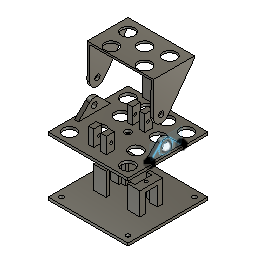
tableXY v18 (Autodesk Fusion 360 design; units mm, degrees)
Autodesk Fusion 360 part; units mm, degrees
sketch "Esquisse2" plane through (0, 0, 0) normal (0, 0, 1) x (1, 0, 0)
  line L0 (-25, 25) -> (25, 25)
  line L1 (25, 25) -> (25, -25)
  line L2 (25, -25) -> (-25, -25)
  line L3 (-25, -25) -> (-25, 25)
  line L4 (-25, 25) -> (25, -25) construction
  line L5 (25, 25) -> (-25, -25) construction
  circle A0 centre (-15.6977, 15.6977) radius 5
  circle A1 centre (-15.6977, -15.6977) radius 5
  circle A2 centre (15.6977, -15.6977) radius 5
  circle A3 centre (15.6977, 15.6977) radius 5
  circle A4 centre (-12.5, 0) radius 5
  circle A5 centre (0, -12.5) radius 5
  circle A6 centre (12.5, 0) radius 5
  circle A7 centre (0, 12.5) radius 5
  dimension "d1" = 50
  dimension "d2" = 50
  dimension "d3" = 10
  dimension "d9" = 360
  dimension "d11" = 10
  dimension "d13" = 360
  constraint horizontal L0
  constraint perpendicular L0 L1
  constraint parallel L0 L2
  constraint parallel L1 L3
  constraint coincident L4 origin
  constraint coincident L5 origin
  constraint coincident L4 A0.centre
  measures "d1" distance of L1.end L2.end
  measures "d2" distance of L0.end L1.end
  measures "d3" diameter of A0
  measures "d11" diameter of A4
extrude "Extrusion1" add sketch "Esquisse2" along normal blind 1.5 makes body 1
sketch "Esquisse3" plane through (0, 0, 0) normal (0, 0, -1) x (1, 0, 0)
  circle A0 centre (-12.5, 0) radius 5
  circle A1 centre (-15.6977, 15.6977) radius 5
  circle A2 centre (15.6977, 15.6977) radius 5
  circle A3 centre (15.6977, -15.6977) radius 5
  circle A4 centre (12.5, 0) radius 5
  circle A5 centre (0, -12.5) radius 5
  circle A6 centre (0, 12.5) radius 5
  circle A7 centre (-15.6977, -15.6977) radius 5
  line L0 (25, 25) -> (-25, 25)
  line L1 (-25, 25) -> (-25, -25)
  line L2 (-25, -25) -> (25, -25)
  line L3 (25, -25) -> (25, 25)
  line L4 (-25, -25) -> (-23, -25)
  line L5 (-23, -25) -> (-23, 25)
  line L6 (-23, 25) -> (-25, 25)
  line L7 (-25, 25) -> (-25, -25)
  line L8 (23, -25) -> (25, -25)
  line L9 (25, -25) -> (25, 25)
  line L10 (25, 25) -> (23, 25)
  line L11 (23, 25) -> (23, -25)
  dimension "d16" = 2
  dimension "d69" = 2
  constraint horizontal L4
  constraint vertical L5
  constraint horizontal L6
  constraint vertical L7
  constraint coincident L1.end L2.start
  constraint horizontal L8
  constraint vertical L9
  constraint horizontal L10
  constraint vertical L11
  constraint coincident L0.start L3.end
  constraint coincident L2 L8.start
  measures "d16" distance of L1.end L4.end
  measures "d69" distance of L9 L11
extrude "Extrusion2" add sketch "Esquisse3" along normal blind 30 contours L0 L2 L3 L8 L9 L10 L11 | L0 L1 L2 L4 L5 L6 L7 bodies 1
sketch "Esquisse4" plane through (-25, 0, 0) normal (-1, 0, 0) x (0, -1, 0)
  line L0 (25, -30) -> (25, 1.5)
  line L1 (25, 1.5) -> (-25, 1.5)
  line L2 (-25, 1.5) -> (-25, -30)
  line L3 (-25, -30) -> (25, -30)
  circle A0 centre (-0.0292, -23.958) radius 5.85
  circle A1 centre (-0.0292, -23.958) radius 2
  line L4 (-25, 0) -> (-4.7346, -27.4339)
  line L5 (5.8207, -23.9237) -> (5.6718, 1.5)
  dimension "d19" = 11.7
  dimension "d20" = 4
  constraint concentric A0 A1
  constraint coincident L2 L4.start
  constraint coincident A0 L4.end
  constraint tangent A0 L4
  constraint coincident A0 L5.start
  constraint coincident L1 L5.end
  constraint tangent A0 L5
  measures "d19" diameter of A0
  measures "d20" diameter of A1
extrude "Extrusion3" cut sketch "Esquisse4" against normal through all contours L0 L1 L2 L3 A0 L4 L5 | A1 bodies 1
sketch "Esquisse8" plane through (23, 0, 0) normal (-1, 0, 0) x (0, -1, 0)
  circle A0 centre (-0.0292, -23.958) radius 2
  line L0 (-4.9916, -14.9971) -> (5.0084, -14.9971)
  line L1 (5.0084, -14.9971) -> (5.0084, 0.0029)
  line L2 (5.0084, 0.0029) -> (-4.9916, 0.0029)
  line L3 (-4.9916, 0.0029) -> (-4.9916, -14.9971)
  line L4 (-4.9916, -14.9971) -> (5.0084, 0.0029) construction
  line L5 (5.0084, -14.9971) -> (-4.9916, 0.0029) construction
  line L6 (-4.9916, 0.0029) -> (-2.9916, 0.0029)
  line L7 (-2.9916, 0.0029) -> (-2.9916, -14.9971)
  line L8 (-2.9916, -14.9971) -> (-4.9916, -14.9971)
  line L9 (-4.9916, -14.9971) -> (-4.9916, 0.0029)
  line L10 (5.0084, 0.0029) -> (3.0084, 0.0029)
  line L11 (3.0084, 0.0029) -> (3.0084, -14.9971)
  line L12 (3.0084, -14.9971) -> (5.0084, -14.9971)
  line L13 (5.0084, -14.9971) -> (5.0084, 0.0029)
  line L14 (5.6806, 0) -> (-25, 0)
  line L15 (-25, 0) -> (-4.7346, -27.4339)
  arc A1 (-4.7346, -27.4339) -> (5.8207, -23.9237) centre (-0.0292, -23.958) ccw
  line L16 (5.8207, -23.9237) -> (5.6806, 0)
  point P0 (0.0084, -7.4971)
  dimension "d28" = 10
  dimension "d29" = 15
  dimension "d30" = 2
  dimension "d31" = 2
  constraint horizontal L0
  constraint perpendicular L0 L1
  constraint parallel L0 L2
  constraint parallel L1 L3
  constraint coincident L4 P0
  constraint coincident L5 P0
  constraint midpoint L5 P0
  constraint horizontal L6
  constraint vertical L7
  constraint horizontal L8
  constraint vertical L9
  constraint horizontal L10
  constraint vertical L11
  constraint horizontal L12
  constraint vertical L13
  measures "d28" distance of L1 L3
  measures "d29" distance of L0 L2
  measures "d30" distance of L2.end L6.end
  measures "d31" distance of L1.end L10.end
extrude "Extrusion4" add sketch "Esquisse8" along normal blind 7 contours L0 L3 L7 L8 L9 L14 | L2 L3 L6 L7 L9 L14 | L0 L1 L11 L12 L13 L14 | L1 L2 L10 L11 L13 L14 bodies 1
fillet "Congé1" radius 2 2 edges at (19.5, 2.9916, -14.9971) (19.5, -3.0084, -14.9971) on bodies 1
ref_plane "Plan de construction1" through (0, 0, -40) normal (0, 0, 1) x (1, 0, 0)
ref_plane "Plan de construction1" through (0, 0, -50) normal (0, 0, 1) x (1, 0, 0) in component "axe vertical"
sketch "Esquisse1" plane through (0, 0, -50) normal (0, 0, 1) x (1, 0, 0) in component "axe vertical"
  line L0 (-30, 30) -> (30, 30)
  line L1 (30, 30) -> (30, -30)
  line L2 (30, -30) -> (-30, -30)
  line L3 (-30, -30) -> (-30, 30)
  line L4 (-30, 30) -> (30, -30) construction
  line L5 (30, 30) -> (-30, -30) construction
  dimension "d39" = 60
  dimension "d40" = 60
  constraint horizontal L0
  constraint perpendicular L0 L1
  constraint parallel L0 L2
  constraint parallel L1 L3
  constraint coincident L4 origin
  constraint coincident L5 origin
  measures "d39" distance of L1.end L2.end
  measures "d40" distance of L0.end L1.end
extrude "Extrusion1'" add sketch "Esquisse1" along normal blind 2 separate body makes body 2 in component "axe vertical"
sketch "Esquisse4 (2)" plane through (0, 0, -48) normal (0, 0, 1) x (-1, 0, 0) in component "axe vertical"
  line L0 (30, 30) -> (-30, 30)
  line L1 (-30, 30) -> (-30, -30)
  line L2 (-30, -30) -> (30, -30)
  line L3 (30, -30) -> (30, 30)
  line L4 (28.2, -12) -> (25.2, -12)
  line L5 (25.2, -12) -> (25.2, 12)
  line L6 (25.2, 12) -> (28.2, 12)
  line L7 (28.2, 12) -> (28.2, -12)
  line L8 (28.2, -12) -> (25.2, 12) construction
  line L9 (25.2, -12) -> (28.2, 12) construction
  line L10 (-25.2, -12) -> (-28.2, -12)
  line L11 (-28.2, -12) -> (-28.2, 12)
  line L12 (-28.2, 12) -> (-25.2, 12)
  line L13 (-25.2, 12) -> (-25.2, -12)
  line L14 (-25.2, -12) -> (-28.2, 12) construction
  line L15 (-28.2, -12) -> (-25.2, 12) construction
  circle A0 centre (22, -22) radius 5
  circle A1 centre (-22, -22) radius 5
  circle A2 centre (22, 22) radius 5
  circle A3 centre (-22, 22) radius 5
  circle A4 centre (8, -22) radius 5
  circle A5 centre (-7, -22) radius 5
  circle A6 centre (-15, 9) radius 5
  circle A7 centre (12.8542, 9.0363) radius 5
  circle A8 centre (13, -8) radius 5
  circle A9 centre (-15, -8) radius 5
  point P0 (26.7, 0)
  point P1 (-26.7, 0)
  dimension "d55" = 3
  dimension "d56" = 24
  dimension "d57" = 25.2
  dimension "d58" = 3
  dimension "d59" = 24
  dimension "d60" = 25.2
  dimension "d166" = 10
  dimension "d167" = 10
  dimension "d168" = 10
  dimension "d169" = 10
  dimension "d170" = 10
  dimension "d171" = 10
  dimension "d174" = 10
  dimension "d175" = 10
  dimension "d176" = 10
  dimension "d177" = 10
  constraint horizontal L4
  constraint perpendicular L4 L5
  constraint parallel L4 L6
  constraint parallel L5 L7
  constraint coincident L8 P0
  constraint coincident L9 P0
  constraint horizontal L10
  constraint perpendicular L10 L11
  constraint parallel L10 L12
  constraint parallel L11 L13
  constraint coincident L14 P1
  constraint coincident L15 P1
  measures "d55" distance of L5.end L6.end
  measures "d56" distance of L4.end L5.end
  measures "d57" distance of origin L5
  measures "d58" distance of L11.end L12.end
  measures "d59" distance of L10.end L11.end
  measures "d60" distance of origin L13
  measures "d166" diameter of A0
  measures "d167" diameter of A1
  measures "d168" diameter of A2
  measures "d169" diameter of A3
  measures "d170" diameter of A4
  measures "d171" diameter of A5
  measures "d174" diameter of A6
  measures "d175" diameter of A7
  measures "d176" diameter of A8
  measures "d177" diameter of A9
extrude "Extrusion14" cut sketch "Esquisse4 (2)" against normal blind 2 contours A0 | A1 | A2 | A3 | A4 | A5 | A6 | A7 | A8 | A9 bodies 2 in component "axe vertical"
extrude "Extrusion3'" add sketch "Esquisse4 (2)" along normal blind 12 contours L4 L5 L6 L7 | L10 L11 L12 L13 bodies 2 in component "axe vertical"
sketch "Esquisse5" plane through (28.2, 0, 0) normal (1, 0, 0) x (0, 1, 0) in component "axe vertical"
  line L0 (-12, -48) -> (12, -48)
  line L1 (12, -48) -> (12, -36)
  line L2 (12, -36) -> (-12, -36)
  line L3 (-12, -36) -> (-12, -48)
  circle A0 centre (-0.0154, -43.1057) radius 2
  circle A1 centre (-0.0154, -43.1057) radius 5
  line L4 (3.5632, -39.6137) -> (12, -48)
  line L5 (-3.4107, -39.4353) -> (-12, -48)
  dimension "d63" = 4
  dimension "d64" = 10
  constraint concentric A0 A1
  constraint coincident A1 L4.start
  constraint coincident L0.end L1.start
  constraint coincident A1 L5.start
  constraint coincident L0.start L3.end
  measures "d63" diameter of A0
  measures "d64" diameter of A1
extrude "Extrusion5" cut sketch "Esquisse5" against normal blind 75 contours L1 L2 L3 A1 L4 L5 | A0 bodies 2 in component "axe vertical"
sketch "Esquisse15" plane through (0, 0, -48) normal (0, 0, 1) x (-1, 0, 0)
  line L0 (30, -30) -> (30, 30)
  line L1 (30, 30) -> (-30, 30)
  line L2 (-30, 30) -> (-30, -30)
  line L3 (-30, -30) -> (30, -30)
  line L4 (28.2, 12) -> (28.2, -12)
  line L5 (28.2, -12) -> (25.2, -12)
  line L6 (25.2, -12) -> (25.2, 12)
  line L7 (25.2, 12) -> (28.2, 12)
  line L8 (-25.2, 12) -> (-25.2, -12)
  line L9 (-25.2, -12) -> (-28.2, -12)
  line L10 (-28.2, -12) -> (-28.2, 12)
  line L11 (-28.2, 12) -> (-25.2, 12)
  line L12 (-6.7, -12) -> (-2.7, -12)
  line L13 (-2.7, -12) -> (-2.7, 23)
  line L14 (-2.7, 23) -> (-6.7, 23)
  line L15 (-6.7, 23) -> (-6.7, -12)
  line L16 (-6.7, -12) -> (-2.7, -12)
  line L17 (-2.7, -12) -> (-2.7, -6)
  line L18 (-2.7, -6) -> (-6.7, -6)
  line L19 (-6.7, -6) -> (-6.7, -12)
  line L20 (-6.7, 23) -> (-2.7, 23)
  line L21 (-2.7, 23) -> (-2.7, 17)
  line L22 (-2.7, 17) -> (-6.7, 17)
  line L23 (-6.7, 17) -> (-6.7, 23)
  line L24 (-6.7, 23) -> (-2.7, 23)
  line L25 (-2.7, 23) -> (-2.7, 17)
  line L26 (-30, 30) -> (-30, -30)
  line L27 (-6.7, -12) -> (-2.7, -12)
  line L28 (-2.7, 23) -> (-6.7, 23)
  line L29 (-2.7, -6) -> (-6.7, -6)
  line L30 (-2.7, -12) -> (-2.7, 23)
  line L31 (-2.7, -12) -> (-2.7, -6)
  line L32 (-2.7, 17) -> (-6.7, 17)
  line L33 (-6.7, -12) -> (-2.7, -12)
  line L34 (-6.7, 17) -> (-6.7, 23)
  line L35 (-6.7, 23) -> (-6.7, -12)
  line L36 (-28.2, 12) -> (-25.2, 12)
  line L37 (-6.7, -6) -> (-6.7, -12)
  line L38 (-25.2, 12) -> (-25.2, -12)
  line L39 (-28.2, -12) -> (-28.2, 12)
  line L40 (-25.2, -12) -> (-28.2, -12)
  line L41 (-2.7, -12) -> (-2.7, 23)
  line L42 (-6.7, 23) -> (-6.7, -12)
  line L43 (-2.7, -12) -> (-2.7, -6)
  line L44 (-6.7, 23) -> (-6.7, -12)
  line L45 (-6.7, -6) -> (-6.7, -12)
  line L46 (-6.7, 17) -> (-6.7, 23)
  line L47 (-6.7, -6) -> (-6.7, -12)
  line L48 (-6.7, 17) -> (-6.7, 23)
  line L49 (-6.7, -12) -> (-2.7, -12)
  line L50 (-2.7, 23) -> (-2.7, 17)
  line L51 (-2.7, 23) -> (-6.7, 23)
  line L52 (-2.7, -12) -> (-2.7, -6)
  line L53 (-2.7, -12) -> (-2.7, 23)
  line L54 (-2.7, 23) -> (-2.7, 17)
  line L55 (-6.7, -12) -> (-2.7, -12)
  line L56 (-6.7, -12) -> (-2.7, -12)
  line L57 (-6.7, 23) -> (-2.7, 23)
  line L58 (-2.7, -6) -> (-6.7, -6)
  line L59 (-2.7, 23) -> (-6.7, 23)
  line L60 (-2.7, 17) -> (-6.7, 17)
  line L61 (-6.7, -12) -> (-2.7, -12)
  line L62 (-2.7, -6) -> (-6.7, -6)
  line L63 (-6.7, 23) -> (-2.7, 23)
  line L64 (-2.7, 17) -> (-6.7, 17)
  line L65 (6.7, -12) -> (6.7, 23)
  line L66 (6.7, -12) -> (6.7, -6)
  line L67 (2.7, 23) -> (2.7, -12)
  line L68 (2.7, -6) -> (2.7, -12)
  line L69 (2.7, 17) -> (2.7, 23)
  line L70 (2.7, -12) -> (6.7, -12)
  line L71 (6.7, 23) -> (2.7, 23)
  line L72 (6.7, 23) -> (6.7, 17)
  line L73 (2.7, -12) -> (6.7, -12)
  line L74 (6.7, -6) -> (2.7, -6)
  line L75 (2.7, 23) -> (6.7, 23)
  line L76 (6.7, 17) -> (2.7, 17)
  circle A0 centre (-22, -22) radius 5
  circle A1 centre (22, -22) radius 5
  circle A2 centre (-22, 22) radius 5
  circle A3 centre (-7, -22) radius 5
  circle A4 centre (8, -22) radius 5
  circle A5 centre (22, 22) radius 5
  circle A6 centre (-15, 9) radius 5
  circle A7 centre (12.8542, 9.0363) radius 5
  circle A8 centre (13, -8) radius 5
  circle A9 centre (-15, -8) radius 5
  point P0 (18, 0)
  dimension "d76" = 4
  dimension "d79" = 6
  dimension "d80" = 6
  dimension "d84" = 4
  dimension "d85" = 35
  dimension "d86" = 6
  dimension "d87" = 6
  dimension "d88" = 6
  dimension "d90" = 4
  dimension "d91" = 35
  dimension "d92" = 6
  dimension "d93" = 6
  dimension "d94" = 6
  dimension "d95" = 4
  dimension "d96" = 35
  dimension "d97" = 6
  dimension "d98" = 6
  dimension "d99" = 6
  dimension "d105" = 4
  dimension "d106" = 35
  dimension "d107" = 6
  dimension "d109" = 6
  dimension "d117" = 18.5
  dimension "d118" = 18.5
  constraint horizontal L12
  constraint vertical L13
  constraint horizontal L14
  constraint vertical L15
  constraint horizontal L16
  constraint vertical L17
  constraint horizontal L18
  constraint vertical L19
  constraint horizontal L20
  constraint vertical L21
  constraint horizontal L22
  constraint vertical L23
  constraint horizontal L27
  constraint vertical L30
  constraint horizontal L28
  constraint vertical L35
  constraint horizontal L33
  constraint vertical L31
  constraint horizontal L29
  constraint vertical L37
  constraint horizontal L24
  constraint vertical L25
  constraint horizontal L32
  constraint vertical L34
  constraint horizontal L61
  constraint vertical L53
  constraint horizontal L59
  constraint vertical L42
  constraint horizontal L56
  constraint vertical L52
  constraint horizontal L58
  constraint vertical L47
  constraint horizontal L57
  constraint vertical L50
  constraint horizontal L60
  constraint vertical L48
  constraint horizontal L55
  constraint vertical L41
  constraint horizontal L51
  constraint vertical L44
  constraint horizontal L49
  constraint vertical L43
  constraint horizontal L62
  constraint vertical L45
  constraint horizontal L63
  constraint vertical L54
  constraint horizontal L64
  constraint vertical L46
  constraint horizontal L73
  constraint vertical L65
  constraint horizontal L71
  constraint vertical L67
  constraint horizontal L70
  constraint vertical L66
  constraint horizontal L74
  constraint vertical L68
  constraint horizontal L75
  constraint vertical L72
  constraint horizontal L76
  constraint vertical L69
  measures "d76" distance of L12.start L12.end
  measures "d79" distance of origin L18
  measures "d80" distance of L14.end L22.end
  measures "d84" distance of L12.end L12.start
  measures "d85" distance of L12.start L14.end
  measures "d86" distance of L18.end L12.start
  measures "d87" distance of origin L29
  measures "d88" distance of L22.end L14.end
  measures "d90" distance of L12.end L12.start
  measures "d91" distance of L12.start L14.end
  measures "d92" distance of L18.end L12.start
  measures "d93" distance of origin L58
  measures "d94" distance of L22.end L14.end
  measures "d95" distance of L12.end L12.start
  measures "d96" distance of L12.start L14.end
  measures "d97" distance of L18.end L12.start
  measures "d98" distance of origin L62
  measures "d99" distance of L22.end L14.end
  measures "d105" distance of L65.start L67.end
  measures "d106" distance of L67.end L67.start
  measures "d107" distance of L68.start L67.end
  measures "d109" distance of L69.start L67.start
  measures "d117" distance of L15 L38
  measures "d118" distance of L6 L65
extrude "Extrusion6" add sketch "Esquisse15" along normal blind 12 contours L12 L13 L15 L16 L17 L18 L19 L27 L29 L30 L31 L33 L35 L37 L41 L42 L43 L44 L45 L47 L49 L52 L53 L55 L56 L58 L61 L62 | L13 L14 L15 L20 L21 L22 L23 L24 L25 L28 L30 L32 L34 L35 L41 L42 L44 L46 L48 L50 L51 L53 L54 L57 L59 L60 L63 L64 | L65 L66 L67 L68 L70 L73 L74 | L65 L67 L69 L71 L72 L75 L76 bodies 2 in component "axe vertical"
sketch "Esquisse16" plane through (-6.7, 0, 0) normal (-1, 0, 0) x (0, -1, 0)
  line L0 (17, -48) -> (23, -48)
  line L1 (23, -48) -> (23, -36)
  line L2 (23, -36) -> (17, -36)
  line L3 (17, -36) -> (17, -48)
  circle A0 centre (-8.2, -42) radius 1.05
  circle A1 centre (19.2, -42) radius 1.05
  line L4 (-6, -48) -> (-6, -36)
  dimension "d111" = 2.1
  dimension "d112" = 2.1
  dimension "d113" = 2.2
  dimension "d114" = 2.2
  measures "d111" diameter of A0
  measures "d112" diameter of A1
  measures "d113" distance of L3 A1.centre
  measures "d114" distance of A0.centre L4
extrude "Extrusion7" cut sketch "Esquisse16" against normal blind 25 contours A0 | A1 bodies 2 in component "axe vertical"
sketch "Esquisse17" plane through (0, 0, -50) normal (0, 0, -1) x (1, 0, 0)
  line L0 (30, 30) -> (-30, 30)
  line L1 (-30, 30) -> (-30, -30)
  line L2 (-30, -30) -> (30, -30)
  line L3 (30, -30) -> (30, 30)
  circle A0 centre (0, 0) radius 1.25
  circle A1 centre (0, 0) radius 2.5
  circle A2 centre (0, 0) radius 5
  circle A3 centre (22, -22) radius 5
  circle A4 centre (-22, -22) radius 5
  circle A5 centre (22, 22) radius 5
  circle A6 centre (7, -22) radius 5
  circle A7 centre (-8, -22) radius 5
  circle A8 centre (-22, 22) radius 5
  circle A9 centre (-12.8542, 9.0363) radius 5
  circle A10 centre (-13, -8) radius 5
  circle A11 centre (15, 9) radius 5
  circle A12 centre (15, -8) radius 5
  dimension "d119" = 2.5
  dimension "d120" = 5
  dimension "d121" = 10
  constraint coincident A0.centre A1.centre
  constraint concentric A0 A2
  measures "d119" diameter of A0
  measures "d120" diameter of A1
  measures "d121" diameter of A2
extrude "Extrusion10" cut sketch "Esquisse17" against normal blind 6.5 contours A0 bodies 2 in component "axe vertical"
extrude "Extrusion9" add sketch "Esquisse17" along normal blind 4.5 contours A1 | A2 bodies 2 in component "axe vertical"
sketch "Esquisse18" plane through (0, 0, -54.5) normal (0, 0, -1) x (1, 0, 0)
  circle A0 centre (0, 0) radius 1.25
  circle A1 centre (0, 0) radius 5
  circle A2 centre (0, 0) radius 2.5
  dimension "d130" = 5
  constraint coincident A0.centre A1.centre
  measures "d130" diameter of A2
extrude "Extrusion12" cut sketch "Esquisse18" against normal blind 2.5 contours A2 bodies 2 in component "axe vertical"
sketch "Esquisse19" plane through (0, 0, -48) normal (0, 0, 1) x (-1, 0, 0)
  circle A0 centre (0, 0) radius 1.25
  line L0 (-2.7, 17) -> (-6.7, 17)
  line L1 (-6.7, 17) -> (-6.7, 23)
  line L2 (-6.7, 23) -> (-2.7, 23)
  line L3 (-2.7, 23) -> (-2.7, 17)
  line L4 (-2.7, -6) -> (-2.7, -12)
  line L5 (-2.7, -12) -> (-6.7, -12)
  line L6 (-6.7, -12) -> (-6.7, -6)
  line L7 (-6.7, -6) -> (-2.7, -6)
  line L8 (6.7, -6) -> (6.7, -12)
  line L9 (6.7, -12) -> (2.7, -12)
  line L10 (2.7, -12) -> (2.7, -6)
  line L11 (2.7, -6) -> (6.7, -6)
  line L12 (6.7, 17) -> (2.7, 17)
  line L13 (2.7, 17) -> (2.7, 23)
  line L14 (2.7, 23) -> (6.7, 23)
  line L15 (6.7, 23) -> (6.7, 17)
  line L16 (30, -30) -> (30, 30)
  line L17 (30, 30) -> (-30, 30)
  line L18 (-30, 30) -> (-30, -30)
  line L19 (-30, -30) -> (30, -30)
  line L20 (28.2, 12) -> (28.2, -12)
  line L21 (28.2, -12) -> (25.2, -12)
  line L22 (25.2, -12) -> (25.2, 12)
  line L23 (25.2, 12) -> (28.2, 12)
  line L24 (-25.2, 12) -> (-25.2, -12)
  line L25 (-25.2, -12) -> (-28.2, -12)
  line L26 (-28.2, -12) -> (-28.2, 12)
  line L27 (-28.2, 12) -> (-25.2, 12)
  circle A1 centre (0, 0) radius 2.5
  circle A2 centre (-22, -22) radius 5
  circle A3 centre (22, -22) radius 5
  circle A4 centre (-22, 22) radius 5
  circle A5 centre (-7, -22) radius 5
  circle A6 centre (8, -22) radius 5
  circle A7 centre (22, 22) radius 5
  circle A8 centre (-15, 9) radius 5
  circle A9 centre (-15, -8) radius 5
  circle A10 centre (12.8542, 9.0363) radius 5
  circle A11 centre (13, -8) radius 5
  dimension "d133" = 5
  constraint concentric A0 A1
  measures "d133" diameter of A1
extrude "Extrusion13" cut sketch "Esquisse19" against normal blind 2 contours A1 bodies 2 in component "axe vertical"
ref_plane "Plan de construction3" through (0, 0, -75) normal (0, 0, -1) x (-1, 0, 0)
sketch "Esquisse1 (2)" plane through (0, 0, -75) normal (0, 0, -1) x (1, 0, 0) in component "socle"
  line L0 (-30, 30, 15.3494) -> (30, 30, 15.3494)
  line L1 (30, 30, 15.3494) -> (30, -30, 15.3494)
  line L2 (30, -30, 15.3494) -> (-30, -30, 15.3494)
  line L3 (-30, -30, 15.3494) -> (-30, 30, 15.3494)
  line L4 (-30, 30, 15.3494) -> (30, -30, 15.3494) construction
  line L5 (30, 30, 15.3494) -> (-30, -30, 15.3494) construction
  dimension "d137" = 60
  dimension "d138" = 60
extrude "Extrusion1''" add sketch "Esquisse1 (2)" along normal blind 2 separate body contours L0 L1 L2 L3 in plane through (0, 0, -90.3494) normal (0, 0, -1) makes body 3 in component "socle"
sketch "Esquisse2 (2)" plane through (0, 0, -90.3494) normal (0, 0, 1) x (1, 0, 0) in component "socle"
  line L0 (30, 30) -> (-30, 30)
  line L1 (-30, 30) -> (-30, -30)
  line L2 (-30, -30) -> (30, -30)
  line L3 (30, -30) -> (30, 30)
  line L4 (17.5, -8.5) -> (-17.5, -8.5)
  line L5 (-17.5, -8.5) -> (-17.5, 8.5)
  line L6 (-17.5, 8.5) -> (17.5, 8.5)
  line L7 (17.5, 8.5) -> (17.5, -8.5)
  line L8 (17.5, -8.5) -> (-17.5, 8.5) construction
  line L9 (-17.5, -8.5) -> (17.5, 8.5) construction
  line L10 (11.5, -6.25) -> (-11.5, -6.25)
  line L11 (-11.5, -6.25) -> (-11.5, 6.25)
  line L12 (-11.5, 6.25) -> (11.5, 6.25)
  line L13 (11.5, 6.25) -> (11.5, -6.25)
  line L14 (11.5, -6.25) -> (-11.5, 6.25) construction
  line L15 (-11.5, -6.25) -> (11.5, 6.25) construction
  line L16 (8, -8.5) -> (-8, -8.5)
  line L17 (-8, -8.5) -> (-8, 8.5)
  line L18 (-8, 8.5) -> (8, 8.5)
  line L19 (8, 8.5) -> (8, -8.5)
  line L20 (8, -8.5) -> (-8, 8.5) construction
  line L21 (-8, -8.5) -> (8, 8.5) construction
  dimension "d141" = 35
  dimension "d142" = 17
  dimension "d143" = 23
  dimension "d144" = 12.5
  dimension "d145" = 16
  dimension "d146" = 17
  constraint horizontal L4
  constraint perpendicular L4 L5
  constraint parallel L4 L6
  constraint parallel L5 L7
  constraint coincident L8 origin
  constraint coincident L9 origin
  constraint horizontal L10
  constraint perpendicular L10 L11
  constraint parallel L10 L12
  constraint parallel L11 L13
  constraint coincident L14 origin
  constraint coincident L15 origin
  constraint horizontal L16
  constraint perpendicular L16 L17
  constraint parallel L16 L18
  constraint parallel L17 L19
  constraint coincident L20 origin
  constraint coincident L21 origin
  measures "d141" distance of L5.end L6.end
  measures "d142" distance of L4.end L5.end
  measures "d143" distance of L11.end L12.end
  measures "d144" distance of L10.end L11.end
  measures "d145" distance of L17.end L18.end
  measures "d146" distance of L16.end L17.end
extrude "Extrusion2'" add sketch "Esquisse2 (2)" along normal blind 17 contours L4 L6 L7 L10 L12 L13 L19 | L4 L5 L6 L10 L11 L12 L17 bodies 3 in component "socle"
sketch "Esquisse3 (2)" plane through (17.5, 0, 0) normal (1, 0, 0) x (0, 1, 0) in component "socle"
  line L0 (-8.5, -90.3494) -> (8.5, -90.3494)
  line L1 (8.5, -90.3494) -> (8.5, -73.3494)
  line L2 (8.5, -73.3494) -> (-8.5, -73.3494)
  line L3 (-8.5, -73.3494) -> (-8.5, -90.3494)
  line L4 (-4.43, -90.3494) -> (4.57, -90.3494)
  line L5 (4.57, -90.3494) -> (4.57, -76.3494)
  line L6 (4.57, -76.3494) -> (-4.43, -76.3494)
  line L7 (-4.43, -76.3494) -> (-4.43, -90.3494)
  line L8 (-4.43, -90.3494) -> (4.57, -76.3494) construction
  line L9 (4.57, -90.3494) -> (-4.43, -76.3494) construction
  point P0 (0.07, -83.3494)
  dimension "d149" = 9
  dimension "d150" = 14
  dimension "d163" = 7
  constraint horizontal L4
  constraint perpendicular L4 L5
  constraint parallel L4 L6
  constraint parallel L5 L7
  constraint coincident L8 P0
  constraint coincident L9 P0
  measures "d149" distance of L5.end L6.end
  measures "d150" distance of L4 L6
  measures "d163" distance of L0 P0
extrude "Extrusion3''" cut sketch "Esquisse3 (2)" against normal blind 40 contours L0 L4 L5 L6 L7 bodies 3 in component "socle"
sketch "Esquisse4 (3)" plane through (0, 0, -73.3494) normal (0, 0, 1) x (-1, 0, 0) in component "socle"
  line L0 (-17.5, -8.5) -> (-8, -8.5)
  line L1 (-8, -8.5) -> (-8, -6.25)
  line L2 (-8, -6.25) -> (-11.5, -6.25)
  line L3 (-11.5, -6.25) -> (-11.5, 6.25)
  line L4 (-11.5, 6.25) -> (-8, 6.25)
  line L5 (-8, 6.25) -> (-8, 8.5)
  line L6 (-8, 8.5) -> (-17.5, 8.5)
  line L7 (-17.5, 8.5) -> (-17.5, -8.5)
  circle A0 centre (-13.6, 0) radius 1.05
  circle A1 centre (13.6, 0) radius 1.05
  dimension "d153" = 2.1
  dimension "d154" = 2.1
  measures "d153" diameter of A0
  measures "d154" diameter of A1
extrude "Extrusion4'" cut sketch "Esquisse4 (3)" against normal blind 10 contours A0 | A1 bodies 3 in component "socle"
sketch "Esquisse5 (2)" plane through (0, 0, -92.3494) normal (0, 0, -1) x (-1, 0, 0) in component "socle"
  line L0 (30, 30) -> (-30, 30)
  line L1 (-30, 30) -> (-30, -30)
  line L2 (-30, -30) -> (30, -30)
  line L3 (30, -30) -> (30, 30)
  circle A0 centre (25, -25) radius 1.5
  circle A1 centre (-25, -25) radius 1.5
  circle A2 centre (25, 25) radius 1.5
  circle A3 centre (-25, 25) radius 1.5
  dimension "d157" = 3
  dimension "d158" = 3
  dimension "d159" = 3
  dimension "d160" = 3
  measures "d157" diameter of A0
  measures "d158" diameter of A1
  measures "d159" diameter of A2
  measures "d160" diameter of A3
extrude "Extrusion5'" cut sketch "Esquisse5 (2)" against normal blind 5 contours A0 | A1 | A2 | A3 bodies 3 in component "socle"
component "axe vertical" placed x (1, 0, 0) y (0, 1, 0) z (0, 0, 1) at (0, 0, 0)
component "socle" placed x (1, 0, 0) y (0, 1, 0) z (0, 0, 1) at (0, 0, 0)
